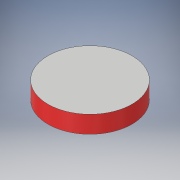
# Autodesk Inventor part: drum
Saved by Autodesk Inventor 2019 (Build 230136000, 136)
## iProperties
Created: 2020-02-08
Part Number: drum
Material: Generic
Document SubType Name: Modeling
Designer: Lenovo
Density: 1 g/cm^3
Appearance: Default
Author: Lenovo
Autodesk Inventor part; units mm, degrees
ref_plane "YZ Plane" through (0, 0, 0) normal (1, 0, 0) x (0, 1, 0)
ref_plane "XZ Plane" through (0, 0, 0) normal (0, 1, 0) x (-1, 0, 0)
ref_plane "XY Plane" through (0, 0, 0) normal (0, 0, 1) x (1, 0, 0)
sketch "Sketch1" plane through (0, 0, 0) normal (0, 1, 0) x (-1, 0, 0)
  circle A0 centre (0, 12.1747) radius 12.108
  arc A1 (7.1431, 10.8771) -> (-7.6488, 10.8771) centre (-0.2529, 11.8554) ccw
  point P0 (0, 0)
  constraints: 2 centre point, 2 point on circle, 1 other
extrude "Extrusion1" add sketch "Sketch1" along normal blind 5
sketch "Sketch2" plane through (0, 0, 12.1747) normal (0, -1, 0) x (1, 0, 0)
  point P0 (0, -12.1747)
sketch "Sketch3" plane through (0, 5, 12.1747) normal (0, 1, 0) x (1, 0, 0)
  point P0 (0, 12.1747)
sketch "Sketch4" plane through (0, 0, 0) normal (0, 1, 0) x (-1, 0, 0)
  arc A0 (2.5285, 18.8375) -> (2.5917, 4.9938) centre (-0.8103, 11.9003) ccw
  point P0 (0, 0)
  constraints: 2 point on circle, 1 centre point, 1 other
scale "Scale1" factors (5, 5, 5) then translate (0, 0, -48.6988) bodies 1
scale "Scale2" factors (2, 2, 2) then translate (0, 0, -12.1747) bodies 1
body "Solid1"
